Autodesk Inventor part; units mm, degrees
(part 5 of 5)
  line L987 (-244.4969, 62.7095) -> (-243.5915, 62.7095)
  line L988 (-243.5915, 62.7095) -> (-243.5915, 62.3643)
  line L989 (-243.5915, 62.3643) -> (-243.583, 62.3643)
  spline S964 degree 2 poles (-243.583, 62.3643) (-243.5321, 62.4549) (-243.3086, 62.6472) (-243.0285, 62.7632) (-242.8644, 62.7632) knots 0 0 0 1 2 3 3 3
  spline S965 degree 2 poles (-242.8644, 62.7632) (-242.6323, 62.7632) (-242.3155, 62.5793) (-242.2108, 62.3813) knots 0 0 0 1 2 2 2
  spline S966 degree 2 poles (-242.2108, 62.3813) (-242.0948, 62.5652) (-241.71, 62.7632) (-241.478, 62.7632) knots 0 0 0 1 2 2 2
  spline S967 degree 2 poles (-241.478, 62.7632) (-241.1328, 62.7632) (-240.7678, 62.3162) (-240.7678, 61.8946) knots 0 0 0 1 2 2 2
  line L990 (-240.7678, 61.8946) -> (-240.7678, 60.5309)
  line L991 (-240.7678, 60.5309) -> (-241.6732, 60.5309)
  line L992 (-239.1495, 60.5309) -> (-239.1495, 60.8619)
  line L993 (-239.1495, 60.8619) -> (-239.158, 60.8619)
  spline S968 degree 2 poles (-239.158, 60.8619) (-239.3758, 60.4772) (-239.8228, 60.4772) knots 0 0 0 1 1 1
  spline S969 degree 2 poles (-239.8228, 60.4772) (-240.1312, 60.4772) (-240.4792, 60.8421) (-240.4792, 61.1505) knots 0 0 0 1 2 2 2
  spline S970 degree 2 poles (-240.4792, 61.1505) (-240.4792, 61.7928) (-239.6899, 61.8946) knots 0 0 0 1 1 1
  line L994 (-239.6899, 61.8946) -> (-239.1495, 61.9654)
  spline S971 degree 2 poles (-239.1495, 61.9654) (-239.1495, 62.0729) (-239.3419, 62.2087) (-239.5031, 62.2087) knots 0 0 0 1 2 2 2
  spline S972 degree 2 poles (-239.5031, 62.2087) (-239.8681, 62.2087) (-240.2755, 61.9993) knots 0 0 0 1 1 1
  line L995 (-240.2755, 61.9993) -> (-240.2755, 62.5878)
  spline S973 degree 2 poles (-240.2755, 62.5878) (-240.1001, 62.6642) (-239.5654, 62.7632) (-239.3758, 62.7632) knots 0 0 0 1 2 2 2
  spline S974 degree 2 poles (-239.3758, 62.7632) (-238.8213, 62.7632) (-238.3205, 62.2879) (-238.3205, 61.7334) knots 0 0 0 1 2 2 2
  line L996 (-238.3205, 61.7334) -> (-238.3205, 60.5309)
  line L997 (-238.3205, 60.5309) -> (-239.1495, 60.5309)
  spline S975 degree 2 poles (-239.687, 61.2722) (-239.687, 61.1845) (-239.5739, 61.0685) (-239.4692, 61.0685) knots 0 0 0 1 2 2 2
  spline S976 degree 2 poles (-239.4692, 61.0685) (-239.3277, 61.0685) (-239.1495, 61.2807) (-239.1495, 61.4476) knots 0 0 0 1 2 2 2
  line L998 (-239.1495, 61.4476) -> (-239.1495, 61.5297)
  line L999 (-239.1495, 61.5297) -> (-239.4579, 61.4872)
  spline S977 degree 2 poles (-239.4579, 61.4872) (-239.687, 61.4476) (-239.687, 61.2722) knots 0 0 0 1 1 1
  line L1000 (-236.5012, 60.5309) -> (-236.5012, 61.7192)
  spline S978 degree 2 poles (-236.5012, 61.7192) (-236.5012, 61.9229) (-236.6229, 62.0984) (-236.7587, 62.0984) knots 0 0 0 1 2 2 2
  spline S979 degree 2 poles (-236.7587, 62.0984) (-236.8747, 62.0984) (-237.0077, 61.9145) (-237.0077, 61.773) knots 0 0 0 1 2 2 2
  line L1001 (-237.0077, 61.773) -> (-237.0077, 60.5309)
  line L1002 (-237.0077, 60.5309) -> (-237.9131, 60.5309)
  line L1003 (-237.9131, 60.5309) -> (-237.9131, 62.7095)
  line L1004 (-237.9131, 62.7095) -> (-237.0077, 62.7095)
  line L1005 (-237.0077, 62.7095) -> (-237.0077, 62.37)
  line L1006 (-237.0077, 62.37) -> (-236.9992, 62.37)
  spline S980 degree 2 poles (-236.9992, 62.37) (-236.8917, 62.5567) (-236.5239, 62.7632) (-236.3088, 62.7632) knots 0 0 0 1 2 2 2
  spline S981 degree 2 poles (-236.3088, 62.7632) (-235.5958, 62.7632) (-235.5958, 61.8607) knots 0 0 0 1 1 1
  line L1007 (-235.5958, 61.8607) -> (-235.5958, 60.5309)
  line L1008 (-235.5958, 60.5309) -> (-236.5012, 60.5309)
  line L1009 (-233.7992, 60.5309) -> (-233.7992, 60.8676)
  line L1010 (-233.7992, 60.8676) -> (-233.8077, 60.8676)
  spline S982 degree 2 poles (-233.8077, 60.8676) (-233.9209, 60.712) (-234.102, 60.5677) (-234.3283, 60.4772) (-234.4783, 60.4772) knots 0 0 0 1 2 3 3 3
  spline S983 degree 2 poles (-234.4783, 60.4772) (-234.8376, 60.4772) (-235.2111, 60.9412) (-235.2111, 61.3939) knots 0 0 0 1 2 2 2
  line L1011 (-235.2111, 61.3939) -> (-235.2111, 62.7095)
  line L1012 (-235.2111, 62.7095) -> (-234.3057, 62.7095)
  line L1013 (-234.3057, 62.7095) -> (-234.3057, 61.4646)
  spline S984 degree 2 poles (-234.3057, 61.4646) (-234.3057, 61.142) (-234.0652, 61.142) knots 0 0 0 1 1 1
  spline S985 degree 2 poles (-234.0652, 61.142) (-233.9322, 61.142) (-233.7992, 61.3175) (-233.7992, 61.4759) knots 0 0 0 1 2 2 2
  line L1014 (-233.7992, 61.4759) -> (-233.7992, 62.7095)
  line L1015 (-233.7992, 62.7095) -> (-232.8939, 62.7095)
  line L1016 (-232.8939, 62.7095) -> (-232.8939, 60.5309)
  line L1017 (-232.8939, 60.5309) -> (-233.7992, 60.5309)
  spline S986 degree 2 poles (-231.6772, 61.3627) (-231.6546, 61.2213) (-231.3773, 61.0628) (-231.151, 61.0628) knots 0 0 0 1 2 2 2
  spline S987 degree 2 poles (-231.151, 61.0628) (-230.8341, 61.0628) (-230.5512, 61.1845) knots 0 0 0 1 1 1
  line L1018 (-230.5512, 61.1845) -> (-230.5512, 60.6101)
  spline S988 degree 2 poles (-230.5512, 60.6101) (-230.8794, 60.4772) (-231.3519, 60.4772) knots 0 0 0 1 1 1
  spline S989 degree 2 poles (-231.3519, 60.4772) (-231.9206, 60.4772) (-232.5543, 61.06) (-232.5543, 61.5721) knots 0 0 0 1 2 2 2
  spline S990 degree 2 poles (-232.5543, 61.5721) (-232.5543, 61.9229) (-232.2771, 62.4577) (-231.731, 62.7632) (-231.4, 62.7632) knots 0 0 0 1 2 3 3 3
  spline S991 degree 2 poles (-231.4, 62.7632) (-231.0633, 62.7632) (-230.5823, 62.5001) (-230.3333, 62.022) (-230.3333, 61.7023) knots 0 0 0 1 2 3 3 3
  line L1019 (-230.3333, 61.7023) -> (-230.3333, 61.3627)
  line L1020 (-230.3333, 61.3627) -> (-231.6772, 61.3627)
  spline S992 degree 2 poles (-231.134, 61.8381) (-231.134, 62.2144) (-231.4028, 62.2144) knots 0 0 0 1 1 1
  spline S993 degree 2 poles (-231.4028, 62.2144) (-231.516, 62.2144) (-231.6688, 62.0078) (-231.6829, 61.8381) knots 0 0 0 1 2 2 2
  line L1021 (-231.6829, 61.8381) -> (-231.134, 61.8381)
  line L1022 (-230.0193, 60.5309) -> (-230.0193, 63.7563)
  line L1023 (-230.0193, 63.7563) -> (-229.1139, 63.7563)
  line L1024 (-229.1139, 63.7563) -> (-229.1139, 60.5309)
  line L1025 (-229.1139, 60.5309) -> (-230.0193, 60.5309)
  spline S994 degree 2 poles (-227.8973, 61.3627) (-227.8746, 61.2213) (-227.5974, 61.0628) (-227.371, 61.0628) knots 0 0 0 1 2 2 2
  spline S995 degree 2 poles (-227.371, 61.0628) (-227.0541, 61.0628) (-226.7712, 61.1845) knots 0 0 0 1 1 1
  line L1026 (-226.7712, 61.1845) -> (-226.7712, 60.6101)
  spline S996 degree 2 poles (-226.7712, 60.6101) (-227.0994, 60.4772) (-227.5719, 60.4772) knots 0 0 0 1 1 1
  spline S997 degree 2 poles (-227.5719, 60.4772) (-228.1406, 60.4772) (-228.7744, 61.06) (-228.7744, 61.5721) knots 0 0 0 1 2 2 2
  spline S998 degree 2 poles (-228.7744, 61.5721) (-228.7744, 61.9229) (-228.4971, 62.4577) (-227.951, 62.7632) (-227.62, 62.7632) knots 0 0 0 1 2 3 3 3
  spline S999 degree 2 poles (-227.62, 62.7632) (-227.2833, 62.7632) (-226.8023, 62.5001) (-226.5534, 62.022) (-226.5534, 61.7023) knots 0 0 0 1 2 3 3 3
  line L1027 (-226.5534, 61.7023) -> (-226.5534, 61.3627)
  line L1028 (-226.5534, 61.3627) -> (-227.8973, 61.3627)
  spline S1000 degree 2 poles (-227.3541, 61.8381) (-227.3541, 62.2144) (-227.6228, 62.2144) knots 0 0 0 1 1 1
  spline S1001 degree 2 poles (-227.6228, 62.2144) (-227.736, 62.2144) (-227.8888, 62.0078) (-227.9029, 61.8381) knots 0 0 0 1 2 2 2
  line L1029 (-227.9029, 61.8381) -> (-227.3541, 61.8381)
  point P0 (0, 0)
  constraints: 8 other
extrude "Estrusione5" cut sketch "Schizzo6" against normal blind 1
